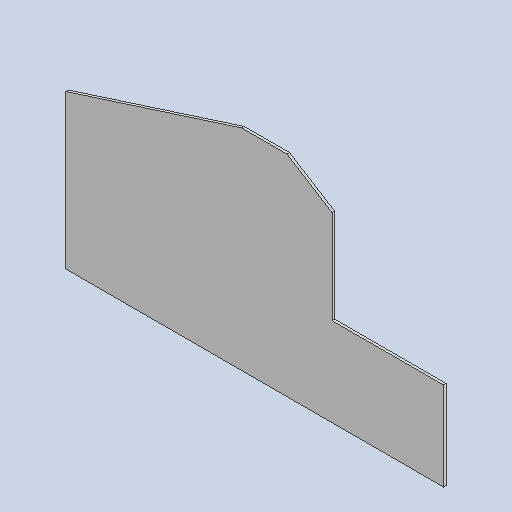
# Autodesk Inventor part: 사이드 카울
Saved by Autodesk Inventor 2025.2 (Build 292293000, 293)
## iProperties
Created: 2025-07-11
Part Number: 사이드 카울
Material: 일반
Document SubType Name: Modeling
Designer: jbhma
Density: 1 g/cm^3
Appearance: 기본값
Author: jbhma
Autodesk Inventor part; units mm, degrees
ref_plane "YZ Plane" through (0, 0, 0) normal (1, 0, 0) x (0, 1, 0)
ref_plane "XZ Plane" through (0, 0, 0) normal (0, 1, 0) x (-1, 0, 0)
ref_plane "XY Plane" through (0, 0, 0) normal (0, 0, 1) x (1, 0, 0)
sketch "스케치4" plane through (0, 0, 0) normal (0, 0, 1) x (1, 0, 0)
  line L0 (0, 0) -> (435, 0)
  line L1 (435, 0) -> (435, 345)
  line L2 (435, 345) -> (0, 345)
  line L3 (0, 0) -> (-1038.851, 0)
  line L4 (-1038.851, 0) -> (-1038.851, 600)
  line L5 (0, 0) -> (-352.5186, 0)
  line L6 (-352.5186, 820) -> (-176.2593, 820)
  line L7 (0, 710) -> (0, 345)
  line L8 (-1038.851, 600) -> (-352.5186, 820)
  line L9 (-176.2593, 820) -> (0, 710)
  dimension "d46" = 435
  dimension "d47" = 1473.851
  dimension "d48" = 345
  dimension "d49" = 475
  dimension "d50" = 435
  dimension "d53" = 787.5186
  dimension "d56" = 600
  constraints: 20 end point, 3 horizontal, 3 parallel, 2 perpendicular
  measures "d46" distance between parallel lines of L1 L7
  measures "d47" distance between parallel lines of L1 L4
  measures "d48" distance between parallel lines of L2 L0
  measures "d49" distance between parallel lines of L2 L6
  measures "d50" distance from line of L0.start L1
  measures "d53" distance from line of L5.end L1
  measures "d56" distance of L3.end L4.end
extrude "돌출3" add sketch "스케치4" along normal blind 10
